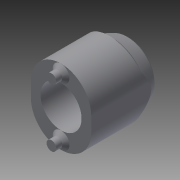
# Autodesk Inventor part: collar
Saved by Autodesk Inventor 2014 (Build 180170000, 170)
## iProperties
Created: 2014-01-14
Part Number: collar
Material: Generic
Document SubType Name: Modeling
Designer: Peele
Density: 1 g/cm^3
Appearance: Default
Author: Peele
Autodesk Inventor part; units mm, degrees
ref_plane "YZ Plane" through (0, 0, 0) normal (1, 0, 0) x (0, 1, 0)
ref_plane "XZ Plane" through (0, 0, 0) normal (0, 1, 0) x (-1, 0, 0)
ref_plane "XY Plane" through (0, 0, 0) normal (0, 0, 1) x (1, 0, 0)
sketch "Sketch1" plane through (0, 0, 0) normal (0, 0, 1) x (1, 0, 0)
  circle A0 centre (0, 0) radius 4.25
  line L0 (0, -1.5) -> (0, 1.5) construction
  line L1 (6.25, -1.5) -> (6.25, 1.5)
  line L2 (-6.25, 1.5) -> (-6.25, -1.5)
  arc A1 (-6.25, -1.5) -> (6.25, -1.5) centre (0, -1.5) ccw
  arc A2 (6.25, 1.5) -> (-6.25, 1.5) centre (0, 1.5) ccw
  dimension "d0" = 8.5
  dimension "d1" = 12.5
  dimension "d2" = 3
  constraints: 8 end point, 4 point on circle, 4 tangent, 3 centre point, 2 coincident, 1 midpoint, 1 parallel, 1 vertical
  measures "d0" diameter of A0
  measures "d1" distance between parallel lines of L1 L2
  measures "d2" distance of L1.start L1.end
extrude "Extrusion1" add sketch "Sketch1" along normal blind 10
sketch "Sketch2" plane through (0, 0, 10) normal (0, 0, 1) x (1, 0, 0)
  circle A0 centre (0, 0) radius 4.25 projected
  line L0 (6.25, -1.5) -> (6.25, 1.5) projected
  line L1 (-6.25, 1.5) -> (-6.25, -1.5) projected
  circle A1 centre (0, 6) radius 1
  circle A2 centre (0, -6) radius 1
  line L2 (0, 6) -> (0, 0) construction
  line L3 (0, 0) -> (0, -6) construction
  dimension "d5" = 2
  dimension "d6" = 6
  constraints: 4 end point, 2 centre point, 2 collinear, 2 parallel, 1 equal radius
  measures "d5" diameter of A1
  measures "d6" distance of L2.start L2.end
extrude "Extrusion2" add sketch "Sketch2" along normal blind 2 contours A1 | A2
sketch "Sketch3" plane through (0, 0, 0) normal (0, 0, -1) x (-1, 0, 0)
  circle A0 centre (0, 0) radius 4.25 projected
  circle A1 centre (0, 0) radius 4.25
  circle A2 centre (0, 0) radius 5.75
  dimension "d9" = 1.5
  constraints: 2 centre point, 2 coincident, 1 concentric
  measures "d9" radial gap between concentric circles of A2 A0
extrude "Extrusion3" add sketch "Sketch3" along normal blind 4
chamfer "Chamfer1" distance 1.95 angle 45 1 edges at (5.75, 0, 0)
chamfer "Chamfer2" distance 1.7 angle 45 1 edges at (5.75, 0, -1.95)
chamfer "Chamfer3" distance 0.35 angle 45 1 edges at (5.75, 0, -4)
chamfer "Chamfer4" distance 0.75 angle 45 2 edges at (-1, -6, 10) (-1, 6, 10)
body "Solid1"
